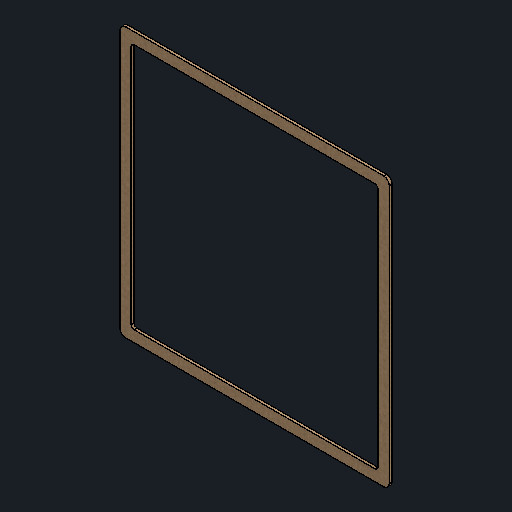
# Autodesk Inventor part: Part1
Saved by Autodesk Inventor 2026.2 (Build 302298000, 298)
## iProperties
Created: 2026-06-15
Part Number: Part1
Material: MDF Medium Density Fiberboard
Document SubType Name: Modeling
Designer: JoshuaEah
Density: 0.8 g/cm^3
Appearance: Cardboard - Corrugated
Author: JoshuaEah
Autodesk Inventor part; units mm, degrees
ref_plane "YZ Plane" through (0, 0, 0) normal (1, 0, 0) x (0, 1, 0)
ref_plane "XZ Plane" through (0, 0, 0) normal (0, 1, 0) x (-1, 0, 0)
ref_plane "XY Plane" through (0, 0, 0) normal (0, 0, 1) x (1, 0, 0)
sketch "Sketch1" plane through (0, 0, 0) normal (0, 0, 1) x (1, 0, 0)
  line L0 (0, 0) -> (304.8, 0)
  line L1 (304.8, 0) -> (304.8, 304.8)
  line L2 (304.8, 304.8) -> (0, 304.8)
  line L3 (0, 304.8) -> (0, 0)
  circle A0 centre (6.35, 298.45) radius 0.9922
  circle A1 centre (298.45, 298.45) radius 0.9922
  circle A2 centre (298.45, 6.35) radius 0.9922
  circle A3 centre (6.35, 6.35) radius 0.9922
  circle A4 centre (6.35, 152.4) radius 0.9922
  circle A5 centre (298.45, 152.4) radius 0.9922
  circle A6 centre (152.4, 298.45) radius 0.9922
  circle A7 centre (152.4, 6.35) radius 0.9922
  line L4 (12.7, 292.1) -> (292.1, 292.1)
  line L5 (292.1, 292.1) -> (292.1, 12.7)
  line L6 (292.1, 12.7) -> (12.7, 12.7)
  line L7 (12.7, 12.7) -> (12.7, 292.1)
  point P0 (304.8, 152.4)
  point P1 (152.4, 304.8)
  dimension "d0" = 304.8
  dimension "d6" = 1.9844
  dimension "d7" = 6.35
  dimension "d8" = 6.35
  dimension "d10" = 6.35
  dimension "d11" = 6.35
  dimension "d19" = 12.7
  dimension "d20" = 12.7
  dimension "d21" = 12.7
  dimension "d22" = 12.7
  constraints: 16 end point, 8 centre point, 7 equal radius, 6 horizontal alignment, 6 vertical alignment, 4 parallel, 3 perpendicular, 2 horizontal, 2 midpoint, 1 coincident
  measures "d0" distance of L1.end L2.end
  measures "d6" diameter of A0
  measures "d7" distance from line of L3 A0.centre
  measures "d8" distance from line of L2 A0.centre
  measures "d10" distance from line of L1 A1.centre
  measures "d11" distance from line of L0 A2.centre
  measures "d19" distance between parallel lines of L3 L7
  measures "d20" distance between parallel lines of L2 L4
  measures "d21" distance between parallel lines of L1 L5
  measures "d22" distance between parallel lines of L0 L6
extrude "Extrusion1" add sketch "Sketch1" against normal blind 3.175 contours L3 L2 L1 L0 | A0 | A1 | A2 | A3 | A4 | A5 | A6 | A7
fillet "Fillet1" radius 6.35 4 edges at (0, 304.8, -1.5875) (304.8, 304.8, -1.5875) (0, 0, -1.5875) (304.8, 0, -1.5875)
fillet "Fillet1" radius 3.175 4 edges at (292.1, 12.7, -1.5875) (292.1, 292.1, -1.5875) (12.7, 292.1, -1.5875) (12.7, 12.7, -1.5875)
equation "\"d10\" = d7"
equation "\"d11\" = d8"
equation "\"d20\" = d19"
equation "\"d21\" = d19"
equation "\"d22\" = d20"
body "Solid1"
